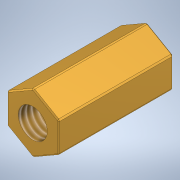
# Autodesk Inventor part: 5002_Brass_Nut_Tx_Rx_Relative_Positioning_MPSv2_v1
Saved by Autodesk Inventor 2021 (Build 250183000, 183)
## iProperties
Created: 2020-11-11
Part Number: 5002_Brass_Nut_Tx_Rx_Relative_Positioning_MPSv2_v1
Material: Brass, Soft Yellow
Document SubType Name: Modeling
Designer: Admin
Density: 8.47 g/cm^3
Appearance: Brass - Satin
Author: Admin
Autodesk Inventor part; units mm, degrees
ref_plane "YZ Plane" through (0, 0, 0) normal (1, 0, 0) x (0, 1, 0)
ref_plane "XZ Plane" through (0, 0, 0) normal (0, 1, 0) x (-1, 0, 0)
ref_plane "XY Plane" through (0, 0, 0) normal (0, 0, 1) x (1, 0, 0)
sketch "Sketch1" plane through (0, 0, 0) normal (0, 0, 1) x (1, 0, 0)
  line L0 (0, 0) -> (0, 6.5)
  line L1 (0, 6.5) -> (5.6292, 3.25)
  line L2 (0, 6.5) -> (6.5, 6.5) construction
  line L3 (5.6292, 3.25) -> (5.6292, -3.25)
  line L4 (5.6292, -3.25) -> (0, -6.5)
  line L5 (0, -6.5) -> (-5.6292, -3.25)
  line L6 (-5.6292, -3.25) -> (-5.6292, 3.25)
  line L7 (-5.6292, 3.25) -> (0, 6.5)
  circle A0 centre (0, 0) radius 3.175
  dimension "d1" = 6.5
  dimension "d2" = 30
  dimension "d3" = 6.35
  constraints: 16 end point, 3 parallel, 2 coincident, 1 centre point, 1 equal length, 1 horizontal, 1 point on line, 1 vertical
  measures "d1" distance of L0.end L1.end
  measures "d2" angle of L1 L2
  measures "d3" diameter of A0
extrude "Extrusion1" add sketch "Sketch1" along normal blind 25
chamfer "Chamfer1" distance 0.25 angle 45 18 edges at (2.8146, 4.875, 25) (5.6292, 0, 25) (2.8146, -4.875, 25) (-2.8146, -4.875, 25) (-5.6292, 0, 25) (-2.8146, 4.875, 25) (0, 6.5, 12.5) (5.6292, 3.25, 12.5) (5.6292, -3.25, 12.5) (0, -6.5, 12.5) (-5.6292, -3.25, 12.5) (-5.6292, 3.25, 12.5) (-2.8146, 4.875, 0) (-5.6292, 0, 0) (-2.8146, -4.875, 0) (2.8146, -4.875, 0) (5.6292, 0, 0) (2.8146, 4.875, 0)
thread "Thread1" size "1/4-20 UNC" class "2B" standard "ANSI Unified Screw Threads" full length
body "Solid1"
